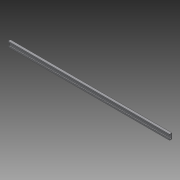
# Autodesk Inventor part: X_Rail-C_shape-Rev1
Saved by Autodesk Inventor 2015 (Build 190159000, 159)
## iProperties
Created: 2016-12-21
Part Number: X_Rail-C_shape-Rev1
Material: Generic
Document SubType Name: Modeling
Designer: Guy
Density: 1 g/cm^3
Appearance: Default
Author: Guy
Autodesk Inventor part; units mm, degrees
ref_plane "YZ Plane" through (0, 0, 0) normal (1, 0, 0) x (0, 1, 0)
ref_plane "XZ Plane" through (0, 0, 0) normal (0, 1, 0) x (-1, 0, 0)
ref_plane "XY Plane" through (0, 0, 0) normal (0, 0, 1) x (1, 0, 0)
sketch "Sketch1" plane through (0, 0, 0) normal (0, 0, 1) x (1, 0, 0)
  line L0 (-30, 0) -> (0, 0)
  line L1 (0, 0) -> (0, 67.45)
  line L2 (0, 67.45) -> (-30, 67.45)
  line L3 (0, 67.45) -> (-30, 67.45)
  line L4 (0, 67.45) -> (0, 0)
  line L5 (0, 0) -> (-30, 0)
  line L6 (-6, 61.45) -> (-24, 61.45)
  line L7 (-6, 6) -> (-6, 61.45)
  line L8 (-30, 51.45) -> (-24, 51.45)
  line L9 (-30, 16) -> (-24, 16)
  line L10 (-24, 6) -> (-24, 16)
  line L11 (-24, 51.45) -> (-24, 61.45)
  line L12 (-30, 0) -> (-30, 16)
  line L13 (-30, 51.45) -> (-30, 67.45)
  line L14 (-24, 6) -> (-6, 6)
  line L15 (-200, 67.45) -> (-200, 61.45)
  dimension "d0" = 67.45
  dimension "d1" = 200
  dimension "d2" = 6
  dimension "d3" = 6
  dimension "d10" = 6
  dimension "d11" = 6
  dimension "d12" = 30
  dimension "d13" = 6
  dimension "d14" = 30
  dimension "d17" = 10
  dimension "d18" = 10
  constraints: 32 end point, 11 parallel, 3 collinear, 3 perpendicular, 2 horizontal, 1 coincident, 1 point on line
  measures "d0" distance of L0.end L1.end
  measures "d1" distance of L1.end L15.start
  measures "d2" distance between parallel lines of L6 L2
  measures "d3" distance between parallel lines of L1 L7
  measures "d10" distance between parallel lines of L11 L13
  measures "d11" distance between parallel lines of L12 L10
  measures "d12" distance between parallel lines of L1 L12
  measures "d13" distance between parallel lines of L0 L14
  measures "d14" distance between parallel lines of L1 L13
  measures "d17" distance between parallel lines of L8 L6
  measures "d18" distance between parallel lines of L14 L9
extrude "Extrusion1" add sketch "Sketch1" along normal blind 2051
body "Solid1"
